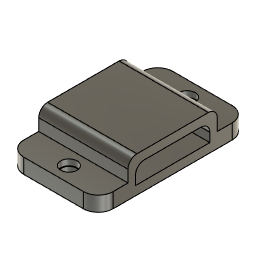
Verrou (Autodesk Fusion 360 design; units mm, degrees)
Autodesk Fusion 360 part; units mm, degrees
sketch "Esquisse1" plane through (0, 0, 0) normal (0, 0, 1) x (1, 0, 0)
  line L0 (10, 25) -> (-10, 25)
  line L1 (-15, 20) -> (-15, -20)
  line L2 (-10, -25) -> (10, -25)
  line L3 (15, -20) -> (15, 20)
  line L4 (15, 25) -> (-15, -25) construction
  line L5 (-15, 25) -> (15, -25) construction
  line L6 (0, 0) -> (0, 40)
  line L7 (0, 40) -> (0, -29.6677)
  circle A0 centre (0, 20) radius 2.5
  circle A1 centre (0, -20) radius 2.5
  arc A2 (-10, 25) -> (-15, 20) centre (-10, 20) ccw
  arc A3 (15, 20) -> (10, 25) centre (10, 20) ccw
  arc A4 (10, -25) -> (15, -20) centre (10, -20) ccw
  arc A5 (-15, -20) -> (-10, -25) centre (-10, -20) ccw
  line L8 (-15, -15) -> (15, -15)
  line L9 (15, -15) -> (15, 15)
  line L10 (15, 15) -> (-15, 15)
  line L11 (-15, 15) -> (-15, -15)
  line L12 (-15, -15) -> (15, 15) construction
  line L13 (15, -15) -> (-15, 15) construction
  line L14 (-15, -12.5) -> (15, -12.5)
  line L15 (15, -12.5) -> (15, 12.5)
  line L16 (15, 12.5) -> (-15, 12.5)
  line L17 (-15, 12.5) -> (-15, -12.5)
  line L18 (-15, -12.5) -> (15, 12.5) construction
  line L19 (15, -12.5) -> (-15, 12.5) construction
  dimension "d1" = 30
  dimension "d2" = 50
  dimension "d3" = 5
  dimension "d4" = 5
  dimension "d5" = 5
  dimension "d6" = 5
  dimension "d7" = 5
  dimension "d8" = 5
  dimension "d9" = 30
  dimension "d10" = 30
  dimension "d20" = 25
  constraint horizontal L0
  constraint perpendicular L0 L1
  constraint parallel L0 L2
  constraint parallel L1 L3
  constraint coincident L4 L6.start
  constraint coincident L5 L6.start
  constraint coincident L6.start origin
  constraint perpendicular L0 L6
  constraint perpendicular L2 L7
  constraint midpoint L6 A0.centre
  constraint coincident L7 A1.centre
  constraint coincident L5.start L1
  constraint coincident L5.start L0
  constraint tangent L1 A2
  constraint tangent L0 A2
  constraint coincident L4.start L3
  constraint coincident L4.start L0
  constraint tangent L3 A3
  constraint tangent L0 A3
  constraint equal A2 A3
  constraint coincident L5.end L3
  constraint coincident L5.end L2
  constraint tangent L3 A4
  constraint tangent L2 A4
  constraint equal A2 A4
  constraint coincident L4.end L2
  constraint coincident L4.end L1
  constraint tangent L2 A5
  constraint tangent L1 A5
  constraint horizontal L8
  constraint perpendicular L8 L9
  constraint parallel L8 L10
  constraint parallel L9 L11
  constraint coincident L12 L6.start
  constraint coincident L13 L6.start
  constraint horizontal L14
  constraint perpendicular L14 L15
  constraint parallel L14 L16
  constraint parallel L15 L17
  constraint coincident L18 L6.start
  constraint coincident L19 L6.start
  constraint coincident L11 L14.start
  measures "d1" distance of L4.end L5.end
  measures "d2" distance of L5.start L4.end
  measures "d3" diameter of A0
  measures "d4" diameter of A1
  measures "d5" distance of L0 A0.centre
  measures "d6" distance of L2 A1.centre
  measures "d7" radius of A2
  measures "d8" radius of A5
  measures "d9" distance of L9.end L10.end
  measures "d10" distance of L8.end L9.end
  measures "d20" distance of L14 L16
extrude "Extrusion1" add sketch "Esquisse1" along normal blind 5 contours L0 L3 L6 L7 A0 A3 L10 | L0 L1 L6 L7 A0 A2 L10 | L2 L3 L7 A1 A4 L8 | L1 L2 L7 A1 A5 L8 makes body 1 at (-9.1574, 21.5425, 0) makes body 2 at (9.1574, -21.5425, 5)
extrude "Extrusion2" add sketch "Esquisse1" along normal blind 12 contours L3 L6 L7 L9 L10 L16 | L3 L6 L7 L9 L14 L15 L16 | L1 L6 L7 L10 L11 L16 | L3 L7 L8 L9 L14 | L1 L6 L7 L11 L14 L16 L17 | L1 L7 L8 L11 L14 bodies 1 2
extrude "Extrusion3" cut sketch "Esquisse1" along normal blind 9 contours L3 L6 L7 L9 L14 L15 L16 | L1 L6 L7 L11 L14 L16 L17 bodies 1
fillet "Congé1" radius 3 2 edges at (0, 15, 12) (0, -15, 12) on bodies 1
delete_face "DeleteFace1" 1 faces at (2.4969, -20.1246, 3.3333) on bodies 1
delete_face "DeleteFace2" 1 faces at (2.4876, 20.2489, 1.6667) on bodies 1
hole "Perçage1" at (0, 19.856, 5) direction (0, 0, -1) diameter 5 depth 5 tip angle 180 counterbore diameter 5.5 counterbore depth 2 bodies 1
hole "Perçage2" at (0, -19.856, 5) direction (0, 0, -1) diameter 5 depth 5 tip angle 180 counterbore diameter 5.5 counterbore depth 2 bodies 1
extrude "Extrusion4" add sketch "Esquisse1" along normal blind 3 contours L3 L6 L7 L9 L14 L15 L16 | L1 L6 L7 L11 L14 L16 L17 bodies 1
fillet "Congé2" radius 3 2 edges at (0, -12.5, 9) (0, 12.5, 9) on bodies 1
